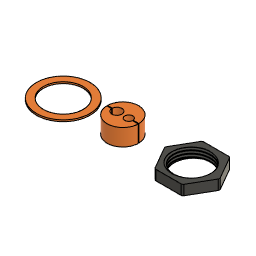
Cable gland accessoires v8 (Autodesk Fusion 360 design; units mm, degrees)
Autodesk Fusion 360 part; units mm, degrees
sketch "Sketch1" plane through (0, 0, 0) normal (0, 0, 1) x (1, 0, 0)
  circle A0 centre (0, 0) radius 7.9
  circle A1 centre (3, 0) radius 2
  circle A2 centre (-3, 0) radius 2.5
  circle A3 centre (0, 0) radius 3 construction
  line L0 (-7.8986, 0.15) -> (-5.4955, 0.15)
  line L1 (4.9944, 0.15) -> (7.8986, 0.15)
  line L2 (-7.8986, -0.15) -> (-5.4955, -0.15)
  line L3 (4.9944, -0.15) -> (7.8986, -0.15)
  line L4 (-7.6392, 0.15) -> (-7.6392, -0.15) construction
  point P0 (-7.6392, 0)
  dimension "d1" = 15.8
  dimension "d2" = 4
  dimension "d4" = 5
  dimension "d5" = 6
  dimension "d7" = 0.3
  constraint coincident A0.centre A3.centre
  constraint coincident A1.centre A3
  constraint horizontal A1.centre A2.centre
  constraint horizontal A0.centre A2.centre
  constraint coincident A2.centre A3
  constraint coincident A0 L0.start
  constraint coincident A2 L0.end
  constraint coincident A1 L1.start
  constraint coincident A0 L1.end
  constraint horizontal L1
  constraint horizontal L0.end L1.start
  constraint coincident A0 L2.start
  constraint coincident A2 L2.end
  constraint horizontal L2
  constraint coincident A1 L3.start
  constraint coincident A0 L3.end
  constraint horizontal L3
  constraint horizontal L2.end L3.start
  constraint coincident L0 L4.start
  constraint coincident L2 L4.end
  constraint perpendicular L2 L4
  constraint midpoint L4 P0
  constraint horizontal A2.centre P0
  constraint horizontal L0
  measures "d1" diameter of A0
  measures "d2" diameter of A1
  measures "d4" diameter of A2
  measures "d5" diameter of A3
  measures "d7" distance of L4.start L4.end
extrude "Extrude1" add sketch "Sketch1" along normal blind 8.5 contours A0 A1 A2 L0 L1 L2 L3 makes body 1
sketch "Sketch2" plane through (0, 0, 0) normal (0, 0, 1) x (1, 0, 0)
  line L0 (56.9033, 12.0029) -> (43.0469, 12.0029)
  line L1 (43.0469, 12.0029) -> (36.1187, 0.0029)
  line L2 (36.1187, 0.0029) -> (43.0469, -11.9971)
  line L3 (43.0469, -11.9971) -> (56.9033, -11.9971)
  line L4 (56.9033, -11.9971) -> (63.8315, 0.0029)
  line L5 (63.8315, 0.0029) -> (56.9033, 12.0029)
  circle A0 centre (49.9751, 0.0029) radius 7.0907
  point P0 (49.9751, 0.0029)
  dimension "d10" = 12
  constraint horizontal L0
  constraint coincident P0 A0.centre
  measures "d10" distance of P0 L5
extrude "Extrude2" add sketch "Sketch2" along normal blind 5 separate body makes body 2
thread "Thread1" "ISO Metric profile 20.0 M20x1.5 6H" major diameter 20.203 minor diameter 18.526 pitch 1.5 angle 60 modelled right hand crest width 0.4065 on face at (57.057, -0.3506, 3.3333) crest through (59.2381, 0.0029, 0.375) on bodies 2
fillet "Fillet1" radius 1 6 edges at (43.0469, -11.9971, 2.5) (36.1187, 0.0029, 2.5) (56.9033, -11.9971, 2.5) (63.8315, 0.0029, 2.5) (56.9033, 12.0029, 2.5) (43.0469, 12.0029, 2.5) on bodies 2
sketch "Sketch3" plane through (0, 0, 0) normal (0, 0, 1) x (1, 0, 0)
  circle A0 centre (-30, 0) radius 10
  circle A1 centre (-30, 0) radius 13.5
  dimension "d15" = 20
  dimension "d16" = 27
  constraint concentric A0 A1
  measures "d15" diameter of A0
  measures "d16" diameter of A1
extrude "Extrude3" add sketch "Sketch3" along normal blind 0.8 separate body makes body 3
copy_body "Body->Comp1" bodies 3 removing the originals makes body 4 in component "seal"
copy_body "Body->Comp2" bodies 1 removing the originals makes body 5 in component "insert"
copy_body "Body->Comp3" bodies 2 removing the originals makes body 6 in component "nut"
move_body "Move1" bodies 6 to x (1, 0, 0) y (0, 1, 0) z (0, 0, 1) at (-15, 0, 0) in component "nut"
component "seal" placed x (1, 0, 0) y (0, 1, 0) z (0, 0, 1) at (0, 0, 0)
component "insert" placed x (1, 0, 0) y (0, 1, 0) z (0, 0, 1) at (0, 0, 0)
component "nut" placed x (1, 0, 0) y (0, 1, 0) z (0, 0, 1) at (0, 0, 0)
equation "d10 = ( 24 / 2 ) * 1 mm"
named bodies: "insert", "nut", "seal"
